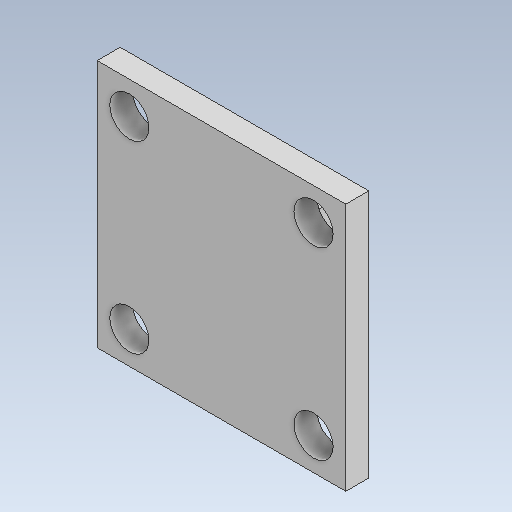
# Autodesk Inventor part: Magazin_1_trichter
Saved by Autodesk Inventor 2025.2 (Build 292293000, 293)
## iProperties
Created: 2025-06-10
Part Number: Magazin_1_trichter
Material: Generisch
Document SubType Name: Modeling
Designer: maria
Density: 1 g/cm^3
Appearance: Vorgabe
Author: maria
## iProperties of the stored document Magazin_1_3D-Druck.ipt
Created: 2025-06-10
Part Number: Magazin_1_3D-Druck
Material: Generisch
Document SubType Name: Modeling
Designer: maria
Density: 1 g/cm^3
Appearance: Vorgabe
Author: maria
Autodesk Inventor part; units mm, degrees
ref_plane "YZ Plane" through (0, 0, 0) normal (1, 0, 0) x (0, 1, 0)
ref_plane "XZ Plane" through (0, 0, 0) normal (0, 1, 0) x (-1, 0, 0)
ref_plane "XY Plane" through (0, 0, 0) normal (0, 0, 1) x (1, 0, 0)
sketch "Skizze1" plane through (0, 0, 0) normal (0, 1, 0) x (-1, 0, 0)
  line L0 (8.2, -1.8) -> (8.2, -14.2)
  line L1 (8.2, -14.2) -> (-0.2, -14.2)
  line L2 (-0.2, -14.2) -> (-0.2, -1.8)
  line L3 (-7, 5) -> (15, 5)
  line L4 (15, 5) -> (15, -21)
  line L5 (15, -21) -> (-7, -21)
  line L6 (-7, -21) -> (-7, 5)
  line L7 (8.2, -1.8) -> (-0.2, -1.8)
  line L8 (13.2, 3.2) -> (-5.2, 3.2)
  line L9 (-5.2, 3.2) -> (-5.2, -19.2)
  line L10 (-5.2, -19.2) -> (13.2, -19.2)
  line L11 (13.2, -19.2) -> (13.2, 3.2)
  point P0 (0, 0)
  point P1 (8, 0)
  point P2 (4, 0)
  point P3 (4, 5)
  point P4 (4, -14.2)
  point P5 (13.2, -8)
  point P6 (8.2, -8)
  point P7 (4, -19.2)
  point P8 (-5.2, -8)
  dimension "d2" = 6.8
  dimension "d3" = 6.8
  dimension "d56" = 26
  dimension "d57" = 22
  dimension "d58" = 6.8
  dimension "d59" = 6.8
  dimension "d61" = 5
  dimension "d62" = 5
  dimension "d63" = 5
  dimension "d65" = 1.8
  dimension "d66" = 0.2
  dimension "d67" = 5
  constraints: 24 end point, 6 midpoint, 5 parallel, 3 perpendicular, 2 horizontal
  measures "d2" distance between parallel lines of L4 L0
  measures "d3" distance between parallel lines of L6 L2
  measures "d56" distance of L3.end L4.end
  measures "d57" distance of L4.end L5.end
  measures "d58" distance between parallel lines of L1 L5
  measures "d59" distance between parallel lines of L3 L7
  measures "d61" distance of point (13.2, -8) point (8.2, -8)
  measures "d62" distance from line of point (4, -19.2) L1
  measures "d63" distance from line of point (-5.2, -8) L2
  measures "d65" vertical distance of L2.end point (0, 0)
  measures "d66" horizontal distance of L2.end point (0, 0)
  measures "d67" distance between parallel lines of L8 L7
extrude "Extrusion1" add sketch "Skizze1" along normal blind 10 contours L11 L10 L9 L8
sketch "Skizze2" plane through (0, 0, 0) normal (0, -1, 0) x (1, 0, 0)
  line L0 (23, 19) -> (-31, 19)
  line L1 (-31, 19) -> (-31, -35)
  line L2 (-31, -35) -> (23, -35)
  line L3 (23, -35) -> (23, 19)
  line L4 (-15, -21) -> (-15, 5) projected
  line L5 (7, -21) -> (-15, -21) projected
  line L6 (7, 5) -> (7, -21) projected
  line L7 (-15, 5) -> (7, 5) projected
  point P0 (0, 0)
  dimension "d11" = 16
  dimension "d12" = 14
  dimension "d13" = 16
  dimension "d14" = 14
  dimension "d35" = 54
  dimension "d36" = 54
  constraints: 8 end point, 2 parallel, 1 horizontal, 1 perpendicular
  measures "d11" distance between parallel lines of L4 L1
  measures "d12" distance between parallel lines of L2 L5
  measures "d13" distance between parallel lines of L3 L6
  measures "d14" distance between parallel lines of L0 L7
  measures "d35" distance of L0.end L1.end
  measures "d36" distance of L0.start L0.end
extrude "Extrusion2" add sketch "Skizze2" along normal blind 5 contours L3 L2 L1 L0 | L4 L7 L6 L5
sketch "Skizze4" plane through (0, 0, 0) normal (0, 1, 0) x (1, 0, 0)
  line L0 (23, 35) -> (23, -19) projected
  line L1 (-31, 35) -> (23, 35) projected
  line L2 (23, -19) -> (-31, -19) projected
  line L3 (-31, -19) -> (-31, 35) projected
  point P0 (0, 0)
  point P1 (16, 28)
  point P2 (16, -12)
  point P3 (-24, -12)
  point P4 (-24, 28)
  dimension "d44" = 7
  dimension "d45" = 7
  dimension "d46" = 7
  dimension "d47" = 7
  dimension "d48" = 7
  dimension "d49" = 7
  dimension "d50" = 7
  dimension "d51" = 7
  dimension "d52" = 40
  dimension "d53" = 40
  dimension "d54" = 40
  dimension "d55" = 40
  measures "d44" distance from line of L0 point (16, 28)
  measures "d45" distance from line of L1 point (16, 28)
  measures "d46" distance from line of L0 point (16, -12)
  measures "d47" distance from line of L2 point (16, -12)
  measures "d48" distance from line of L3 point (-24, -12)
  measures "d49" distance from line of L2 point (-24, -12)
  measures "d50" distance from line of L1 point (-24, 28)
  measures "d51" distance from line of L3 point (-24, 28)
  measures "d52" distance of point (16, -12) point (16, 28)
  measures "d53" distance of point (-24, 28) point (16, 28)
  measures "d54" distance of point (-24, -12) point (-24, 28)
  measures "d55" distance of point (16, -12) point (-24, -12)
hole "Bohrung1" at (16, 0, -28) at (16, 0, 12) at (-24, 0, 12) at (-24, 0, -28) direction (0, -1, 0) diameter 8.5 depth 5
chamfer "Fasen5" distance 10 angle 21.8 1 edges at (-8.2, 10, -8) measured on face at (-8.2, 3.3333, -5.9333)
chamfer "Fasen6" distance 10 angle 21.8 1 edges at (-4, 10, -1.8) measured on face at (-2.6, 3.3335, -1.8)
chamfer "Fasen7" distance 10 angle 21.8 1 edges at (0.2, 10, -8) measured on face at (0.2, 3.3335, -10.0667)
chamfer "Fasen8" distance 10 angle 21.8 1 edges at (-4, 10, -14.2) measured on face at (-2.6, 6.6668, -14.2)
